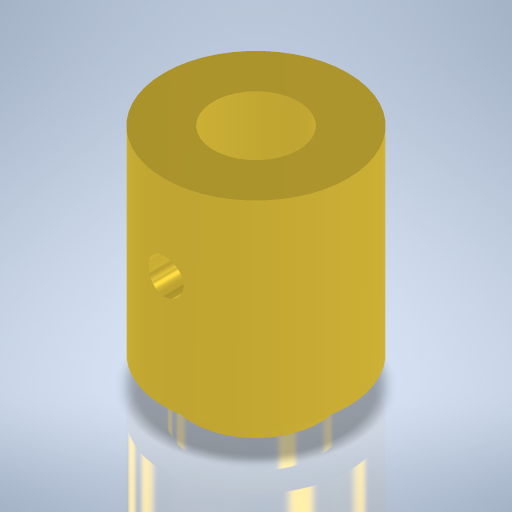
# Autodesk Inventor part: 205 part 2
Saved by Autodesk Inventor 2024 (Build 280153000, 153)
## iProperties
Created: 2024-07-12
Part Number: 205 part 2
Material: Gold
Document SubType Name: Modeling
Designer: ffogue
Density: 19.3 g/cm^3
Appearance: Metall - 2400F (heiß)
Author: ffogue
Autodesk Inventor part; units mm, degrees
ref_plane "YZ Plane" through (0, 0, 0) normal (1, 0, 0) x (0, 1, 0)
ref_plane "XY Plane" through (0, 0, 0) normal (0, 0, 1) x (1, 0, 0)
sketch "Skizze1" plane through (0, 0, 0) normal (0, 1, 0) x (-1, 0, 0)
  line L0 (0, 0) -> (6.5, 0)
  line L1 (6.5, 0) -> (6.5, -14)
  line L2 (6.5, -14) -> (0, -14)
  line L3 (0, -14) -> (0, 0)
  point P0 (6.5, -7)
  dimension "d0" = 13
  dimension "d1" = 14
  constraints: 8 end point, 3 perpendicular, 1 horizontal, 1 midpoint
  measures "d0" diameter of point (6.5, -7) L3
  measures "d1" distance between parallel lines of L2 L0
revolve "Umdrehung1" add sketch "Skizze1" angle 360 about axis through (0, 0, -14) along (0, 0, 1)
ref_plane "Arbeitsebene1" through (0, 6.5, 0) normal (0, 1, 0) x (-1, 0, 0)
sketch "Skizze3" plane through (0, 6.5, 0) normal (0, 1, 0) x (-1, 0, 0)
  point P0 (0, 0)
  point P1 (0, -6)
  dimension "d11" = 6
  constraints: 1 vertical alignment
  measures "d11" distance of point (0, -6) point (0, 0)
hole "Bohrung2" at (0, 6.5, -6) direction (0, -1, 0) diameter 2.5 end through all
sketch "Skizze6" plane through (0, 0, -14) normal (0, 0, -1) x (-1, 0, 0)
  circle A0 centre (0, 0) radius 4.5
  point P0 (0, 0)
  constraints: 1 centre point
extrude "Extrusion1" add sketch "Skizze6" along normal blind 2
sketch "Skizze4" plane through (0, 0, 0) normal (0, 0, 1) x (1, 0, 0)
  circle A0 centre (0, 0) radius 6.5 projected
  point P0 (0, 0)
  constraints: 1 coincident
hole "Bohrung3" at (0, 0, 0) direction (0, 0, -1) diameter 6 end through all
